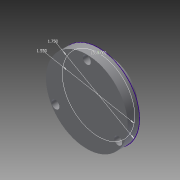
# Autodesk Inventor part: 7.1 Q6
Saved by Autodesk Inventor 2015 (Build 190159000, 159)
## iProperties
Created: 2018-02-08
Part Number: 7.1 Q6
Material: Generic
Document SubType Name: Modeling
Designer: Administrator
Density: 1 g/cm^3
Appearance: Default
Author: Administrator
Autodesk Inventor part; units mm, degrees
ref_plane "YZ Plane" through (0, 0, 0) normal (1, 0, 0) x (0, 1, 0)
ref_plane "XZ Plane" through (0, 0, 0) normal (0, 1, 0) x (-1, 0, 0)
ref_plane "XY Plane" through (0, 0, 0) normal (0, 0, 1) x (1, 0, 0)
sketch "Sketch1" plane through (0, 0, 0) normal (0, 0, 1) x (1, 0, 0)
  circle A0 centre (0, 0) radius 22.225
  circle A1 centre (0, 0) radius 19.685 construction
  circle A2 centre (0, 0) radius 19.685 construction
  circle A3 centre (0, 0) radius 19.685 construction
  point P0 (0, 19.685)
  point P1 (-17.0477, -9.8425)
  point P2 (17.0477, -9.8425)
  dimension "d1" = 39.37
  dimension "d0" = 44.45
  dimension "d4" = 360
  constraints: 4 coincident, 1 centre point, 1 vertical alignment, 16 other
  measures "d0" diameter of A0
extrude "Extrusion1" add sketch "Sketch1" along normal blind 6.35
sketch "Sketch2" plane through (0, 0, 0) normal (0, 0, -1) x (-1, 0, 0)
  circle A0 centre (0, 0) radius 14.7955
  dimension "d8" = 29.591
  constraints: 1 centre point, 1 coincident
  measures "d8" diameter of A0
extrude "Extrusion2" add sketch "Sketch2" along normal blind 6.35
hole "Hole1" at (0, 19.685, 0) at (-17.0477, -9.8425, 0) at (17.0477, -9.8425, 0) direction (0, 0, 1) diameter 4.3688 end through all
body "Solid1"
